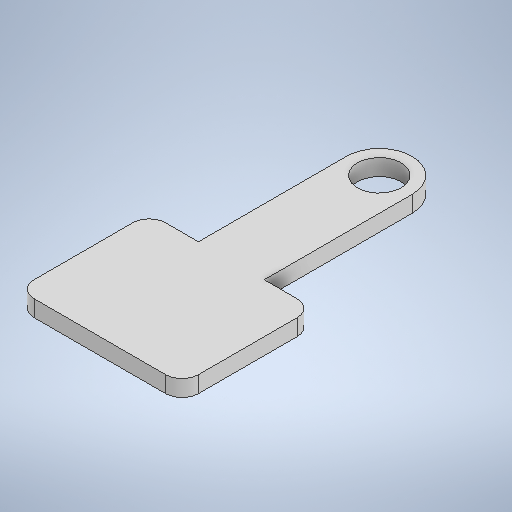
# Autodesk Inventor part: Pomodoro Robot Servo's piece
Saved by Autodesk Inventor 2025.3 (Build 293356030, 356C)
## iProperties
Created: 2026-07-20
Part Number: Pomodoro Robot Servo's piece
Material: Generic
Document SubType Name: Modeling
Designer: Samuel Correa Vega
Density: 1 g/cm^3
Appearance: Default
Author: Samuel Correa Vega
Autodesk Inventor part; units mm, degrees
ref_plane "YZ Plane" through (0, 0, 0) normal (1, 0, 0) x (0, 1, 0)
ref_plane "XZ Plane" through (0, 0, 0) normal (0, 1, 0) x (-1, 0, 0)
ref_plane "XY Plane" through (0, 0, 0) normal (0, 0, 1) x (1, 0, 0)
sketch "Sketch1" plane through (0, 0, 0) normal (0, 1, 0) x (-1, 0, 0)
  arc A0 (-3.2658, -7.0635) -> (4, -4.7538) centre (0, -4.7538) ccw
  arc A1 (-4, -4.7538) -> (-3.2658, -7.0635) centre (0, -4.7538) ccw
  line L0 (4, -4.7538) -> (4, 13.2462)
  line L1 (4, 13.2462) -> (8, 13.2462)
  line L2 (10, 15.2462) -> (10, 27.2462)
  line L3 (8, 29.2462) -> (-8, 29.2462)
  line L4 (-10, 27.2462) -> (-10, 15.2462)
  line L5 (-8, 13.2462) -> (-4, 13.2462)
  line L6 (-4, 13.2462) -> (-4, -4.7538)
  circle A2 centre (0, -4.7538) radius 2.65
  arc A3 (8, 13.2462) -> (10, 15.2462) centre (8, 15.2462) ccw
  arc A4 (10, 27.2462) -> (8, 29.2462) centre (8, 27.2462) ccw
  arc A5 (-8, 29.2462) -> (-10, 27.2462) centre (-8, 27.2462) ccw
  arc A6 (-10, 15.2462) -> (-8, 13.2462) centre (-8, 15.2462) ccw
  point P0 (0, 0)
  point P1 (0, 29.2462)
  dimension "d1" = 4
  dimension "d2" = 5.3
  dimension "d6" = 2
  dimension "d7" = 2
  dimension "d9" = 20
  dimension "d10" = 16
  dimension "d13" = 18
  constraints: 14 end point, 12 point on circle, 9 tangent, 7 centre point, 6 perpendicular, 2 equal radius, 2 vertical alignment, 1 coincident, 1 concentric, 1 horizontal alignment, 1 midpoint, 1 parallel, 1 vertical
  measures "d1" radius of A0
  measures "d2" diameter of A2
  measures "d6" radius of A3
  measures "d7" radius of A4
  measures "d9" distance between parallel lines of L4 L2
  measures "d10" distance between parallel lines of L3 L1
  measures "d13" distance of L5.end L6.end
extrude "Extrusion2" add sketch "Sketch1" along normal blind 2
body "Solid2"
